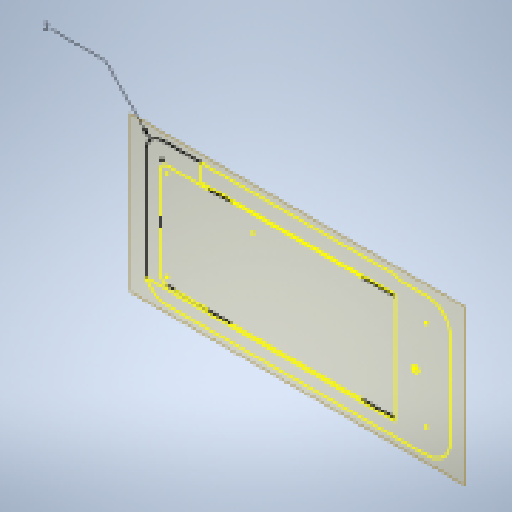
# Autodesk Inventor part: ServoPlate
Saved by Autodesk Inventor 2024.2 (Build 282272000, 272)
## iProperties
Created: 2024-03-19
Part Number: ServoPlate
Material: Ogólny
Document SubType Name: Modeling
Designer: Daniel
Density: 1 g/cm^3
Appearance: Domyślna
Author: Daniel
Autodesk Inventor part; units mm, degrees
ref_plane "YZ Plane" through (0, 0, 0) normal (1, 0, 0) x (0, 1, 0)
ref_plane "XZ Plane" through (0, 0, 0) normal (0, 1, 0) x (-1, 0, 0)
ref_plane "XY Plane" through (0, 0, 0) normal (0, 0, 1) x (1, 0, 0)
ref_plane "Płaszczyzna konstrukcyjna1" through (0, 0, 0) normal (0, 0, 1) x (1, 0, 0)
sketch "Szkic1" plane through (0, 0, 0) normal (0, 0, 1) x (1, 0, 0)
  line L0 (23.2, 1) -> (23.2, -9.5) projected
  arc A0 (23.2, 1) -> (20.35, 3.85) centre (20.35, 1) ccw projected
  line L1 (20.35, 3.85) -> (17.375, 3.85) projected
  line L2 (17.375, 3.85) -> (16.7, 4.15) projected
  line L3 (16.7, 4.15) -> (-6.1, 4.15) projected
  line L4 (-6.1, 4.15) -> (-6.1, 2.15) projected
  line L5 (16.7, 2.15) -> (-6.1, 2.15) projected
  line L6 (16.7, -10.75) -> (16.7, 2.15) projected
  line L7 (16.7, -10.75) -> (-12.6112, -10.75) projected
  arc A1 (-12.6112, -10.75) -> (-10.05, -12.35) centre (-10.05, -9.5) ccw projected
  line L8 (-10.05, -12.35) -> (20.35, -12.35) projected
  arc A2 (20.35, -12.35) -> (23.2, -9.5) centre (20.35, -9.5) ccw projected
  circle A3 centre (19.05, -4.25) radius 0.4 projected
  line L9 (-5.25, 1.85) -> (-10.05, 1.85) projected
  line L10 (-10.9, 1) -> (-10.9, -3.7) projected
  arc A4 (-10.05, 1.85) -> (-10.9, 1) centre (-10.05, 1) ccw projected
  line L11 (-10.9, -4.8) -> (-10.9, -9.5) projected
  arc A5 (-10.9, -9.5) -> (-10.05, -10.35) centre (-10.05, -9.5) ccw projected
  line L12 (-10.05, -10.35) -> (-5.25, -10.35) projected
  line L13 (-12.6112, -10.75) -> (-12.6112, 2.15)
  line L14 (-10.6112, 4.15) -> (-6.1, 4.15)
  arc A6 (-10.6112, 4.15) -> (-12.6112, 2.15) centre (-10.6112, 2.15) ccw
  line L15 (-2.55, 1.95) -> (12.85, 1.95) projected
  line L16 (12.85, -10.45) -> (-2.55, -10.45) projected
  line L17 (-2.55, -10.45) -> (-10.05, -10.35)
  line L18 (12.85, -10.45) -> (16.7, -10.45)
  line L19 (12.85, 1.95) -> (16.7, 1.95)
  line L20 (-2.55, 1.95) -> (-5.25, 1.85)
  line L21 (-10.9, -3.7) -> (-10.9, -4.8)
  line L22 (16.3, 1) -> (16.3, -9.5) projected
  arc A7 (15.55, -10.25) -> (16.3, -9.5) centre (15.55, -9.5) ccw projected
  line L23 (15.55, -10.25) -> (-5.25, -10.25) projected
  arc A8 (-6, -9.5) -> (-5.25, -10.25) centre (-5.25, -9.5) ccw projected
  line L24 (-6, -9.5) -> (-6, 1) projected
  arc A9 (-5.25, 1.75) -> (-6, 1) centre (-5.25, 1) ccw projected
  line L25 (-5.25, 1.75) -> (15.55, 1.75) projected
  arc A10 (16.3, 1) -> (15.55, 1.75) centre (15.55, 1) ccw projected
  line L26 (-1.9, -0.65) -> (1.2, -0.65) projected
  line L27 (-1.9, -1.75) -> (-1.9, -0.65) projected
  line L28 (1.2, -1.75) -> (-1.9, -1.75) projected
  line L29 (1.2, -0.65) -> (1.2, -1.75) projected
  line L30 (5.4, 0.75) -> (5.4, 0.4385) projected
  arc A11 (5.4, 0.75) -> (5.4, -2.85) centre (5.8571, -1.05) ccw projected
  line L31 (5.4, -2.5385) -> (5.4, -2.85) projected
  arc A12 (4.3078, -1.2057) -> (5.4, -2.5385) centre (5.8571, -1.05) ccw projected
  line L32 (5.4, -1.2057) -> (4.3078, -1.2057) projected
  line L33 (5.4, -0.8943) -> (5.4, -1.2057) projected
  line L34 (4.3078, -0.8943) -> (5.4, -0.8943) projected
  arc A13 (5.4, 0.4385) -> (4.3078, -0.8943) centre (5.8571, -1.05) ccw projected
  line L35 (3.9, 0.75) -> (3.9, 0.4385) projected
  arc A14 (3.9, 0.75) -> (3.9, -2.85) centre (4.3571, -1.05) ccw projected
  line L36 (3.9, -2.5385) -> (3.9, -2.85) projected
  arc A15 (3.9, 0.4385) -> (3.9, -2.5385) centre (4.3571, -1.05) ccw projected
  circle A16 centre (-4.75, -8.6) radius 1 projected
  circle A17 centre (15.05, -8.6) radius 1 projected
  circle A18 centre (15.05, 0.1) radius 1 projected
  circle A19 centre (-4.75, 0.1) radius 1 projected
  line L37 (10.7377, -7.5396) -> (10.2468, -7.5396) projected
  line L38 (10.2468, -7.5396) -> (10.2468, -7.75) projected
  line L39 (10.2468, -7.75) -> (11.4156, -7.75) projected
  line L40 (11.4156, -7.75) -> (11.4156, -7.5396) projected
  line L41 (11.4156, -7.5396) -> (10.9247, -7.5396) projected
  line L42 (10.9247, -7.5396) -> (10.9247, -5.95) projected
  line L43 (10.9247, -5.95) -> (10.7377, -5.95) projected
  line L44 (10.7377, -5.95) -> (10.7377, -7.5396) projected
  line L45 (11.626, -7.75) -> (12.1804, -7.75) projected
  spline S0 degree 3 poles (12.1804, -7.75) (12.1963, -7.75) (12.2267, -7.75) (12.2708, -7.7479) (12.3118, -7.7457) (12.3495, -7.7415) (12.384, -7.7369) (12.4153, -7.7312) (12.4433, -7.7239) (12.4607, -7.7181) (12.469, -7.7153) knots 0 0 0 0 0.162643 0.312901 0.453294 0.58413 0.70285 0.811058 0.910586 1 1 1 1 projected
  spline S1 degree 3 poles (12.469, -7.7153) (12.4794, -7.7113) (12.5003, -7.7032) (12.5297, -7.6872) (12.5577, -7.6693) (12.5841, -7.6488) (12.6087, -7.6256) (12.6318, -7.6) (12.653, -7.5717) (12.6725, -7.5411) (12.6907, -7.5086) (12.7057, -7.4738) (12.7192, -7.4375) (12.7294, -7.3991) (12.7381, -7.3591) (12.7436, -7.3172) (12.7476, -7.2734) (12.7479, -7.2436) (12.7481, -7.2284) knots 0 0 0 0 0.056072 0.112012 0.167171 0.222811 0.27891 0.336355 0.395158 0.456072 0.518045 0.581404 0.645662 0.712108 0.780061 0.850885 0.92373 1 1 1 1 projected
  spline S2 degree 3 poles (12.7481, -7.2284) (12.7477, -7.2084) (12.7471, -7.1693) (12.7412, -7.1122) (12.7313, -7.058) (12.7179, -7.0065) (12.7004, -6.9578) (12.6787, -6.912) (12.6533, -6.8689) (12.6243, -6.8285) (12.5902, -6.7918) (12.5498, -6.7603) (12.5042, -6.7334) (12.4527, -6.7121) (12.3959, -6.6948) (12.3332, -6.683) (12.2648, -6.6762) (12.2175, -6.6752) (12.1929, -6.6747) knots 0 0 0 0 0.066633 0.130318 0.191414 0.250222 0.307644 0.363778 0.418941 0.474177 0.529339 0.585724 0.64416 0.705484 0.771261 0.841987 0.917917 1 1 1 1 projected
  line L46 (12.1929, -6.6747) -> (11.813, -6.6747) projected
  line L47 (11.813, -6.6747) -> (11.813, -5.95) projected
  line L48 (11.813, -5.95) -> (11.626, -5.95) projected
  line L49 (11.626, -5.95) -> (11.626, -7.75) projected
  line L50 (-2.2056, -2.52) -> (-2.1, -2.4134) projected
  line L51 (-0.9587, -3.7548) -> (-2.2056, -2.52) projected
  line L52 (-1.121, -5.7025) -> (-0.9587, -3.7548) projected
  line L53 (-2.2056, -6.7765) -> (-1.121, -5.7025) projected
  line L54 (-2.1, -6.8831) -> (-2.2056, -6.7765) projected
  line L55 (-1.1402, -5.9326) -> (-2.1, -6.8831) projected
  line L56 (-1.1875, -6.5) -> (-1.1402, -5.9326) projected
  line L57 (-1.1875, -6.5) -> (-1.5, -6.5) projected
  line L58 (-1.5, -6.65) -> (-1.5, -6.5) projected
  line L59 (-1.2, -6.65) -> (-1.5, -6.65) projected
  arc A20 (-1.2, -6.65) -> (1.2, -6.65) centre (0, -5.75) ccw projected
  line L60 (1.2, -6.65) -> (1.2, -6.15) projected
  line L61 (1.2, -6.15) -> (1.4598, -6.15) projected
  line L62 (2.2, -6.8831) -> (1.4598, -6.15) projected
  line L63 (2.3056, -6.7765) -> (2.2, -6.8831) projected
  line L64 (1.6, -6.0778) -> (2.3056, -6.7765) projected
  line L65 (1.6, -6.0778) -> (1.6, -5.45) projected
  line L66 (1.2, -5.45) -> (1.6, -5.45) projected
  line L67 (1.2, -5.45) -> (1.2, -3.6149) projected
  line L68 (2.3056, -2.52) -> (1.2, -3.6149) projected
  line L69 (2.2, -2.4134) -> (2.3056, -2.52) projected
  line L70 (1.3978, -3.2079) -> (2.2, -2.4134) projected
  arc A21 (1.3978, -3.2079) -> (0.6536, -3.05) centre (1, -3.25) ccw projected
  line L71 (0.6536, -3.05) -> (-0.75, -3.05) projected
  line L72 (-0.75, -3.05) -> (-0.75, -2.75) projected
  line L73 (-0.9, -2.75) -> (-0.75, -2.75) projected
  line L74 (-0.9, -3.05) -> (-0.9, -2.75) projected
  line L75 (-0.9425, -3.5598) -> (-0.9, -3.05) projected
  line L76 (-2.1, -2.4134) -> (-0.9425, -3.5598) projected
  point P0 (0, 0)
  point P1 (-12.6112, 4.15)
  dimension "d0" = 2
  constraints: 14 end point, 5 point on line, 3 perpendicular, 2 collinear, 2 point on circle, 2 tangent, 1 centre point
  measures "d0" radius of A6
extrude "Wyciągnięcie proste1" add sketch "Szkic1" along normal blind 4 contours L0 A2 L8 A1 L7 L6 L5 L4 L3 L2 L1 A0 | L13 A6 L14 L4 L5 L6 L19 L15 L20 L9 A4 L10 L21 L11 A5 L17 L16 L18 L7 | L18 L16 L17 A5 L11 L21 L10 A4 L9 L20 L15 L19 L6
